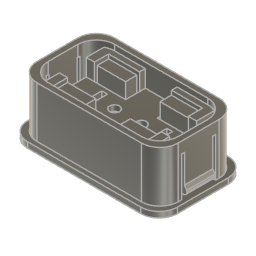
miata-dash-clip (Autodesk Fusion 360 design; units mm, degrees)
Autodesk Fusion 360 part; units mm, degrees
other "Grundnetzelement1"
sketch "Skizze1" plane through (0, 0, 0) normal (0, 0, 1) x (1, 0, 0)
  line L0 (0, 0) -> (53, 0)
  line L1 (53, 0) -> (53, 31)
  line L2 (53, 31) -> (0, 31)
  line L3 (0, 31) -> (0, 0)
  line L4 (1.5, 29.2511) -> (51.4995, 29.2511)
  line L5 (51.4995, 29.2511) -> (51.4995, 1.752)
  line L6 (51.4995, 1.752) -> (1.5, 1.752)
  line L7 (1.5, 1.752) -> (1.5, 29.2511)
  line L8 (49.4995, 27.2511) -> (49.4995, 3.752)
  line L9 (49.4995, 3.752) -> (3.5, 3.752)
  line L10 (3.5, 3.752) -> (3.5, 27.2511)
  line L11 (3.5, 27.2511) -> (49.4995, 27.2511)
  dimension "d1" = 2
  constraint horizontal L0
  constraint vertical L1
  constraint horizontal L2
  constraint vertical L3
  constraint coincident L0.start L3.end
  constraint horizontal L4
  constraint vertical L5
  constraint horizontal L6
  constraint vertical L7
extrude "Extrusion1" add sketch "Skizze1" along normal blind 2 contours L0 L1 L2 L3 | L4 L5 L6 L7 makes body 1
extrude "Extrusion2" add sketch "Skizze1" along normal blind 20 contours L4 L5 L6 L7 bodies 1
fillet "Abrundung1" radius 6.5 12 edges at (51.4995, 29.2511, 11) (53, 31, 1) (53, 0, 1) (51.4995, 1.752, 11) (0, 0, 1) (1.5, 1.752, 11) (0, 31, 1) (1.5, 29.2511, 11) (49.4995, 27.2511, 10) (3.5, 27.2511, 10) (3.5, 3.752, 10) (49.4995, 3.752, 10) on bodies 1
sketch "Skizze2" plane through (51.4995, 0, 0) normal (1, 0, 0) x (0, 1, 0)
  line L0 (8.252, 20) -> (8.252, 2)
  line L1 (8.252, 2) -> (22.7511, 2)
  line L2 (22.7511, 2) -> (22.7511, 20)
  line L3 (22.7511, 20) -> (8.252, 20)
  line L4 (10.5, 16) -> (9.5, 16)
  line L5 (9.5, 16) -> (9.5, 2)
  line L6 (10.5, 16) -> (10.5, 3)
  line L7 (10.5, 3) -> (20.5, 3)
  line L8 (20.5, 3) -> (20.5, 16)
  line L9 (20.5, 16) -> (21.5, 16)
  line L10 (21.5, 16) -> (21.5, 2)
  constraint horizontal L4
  constraint coincident L1 L5.end
  constraint perpendicular L1 L5
  constraint perpendicular L4 L6
  constraint perpendicular L6 L7
  constraint perpendicular L7 L8
  constraint perpendicular L8 L9
  constraint coincident L1 L10.end
  constraint perpendicular L1 L10
extrude "Extrusion3" cut sketch "Skizze2" against normal blind 58 contours L1 L4 L5 L6 L7 L8 L9 L10 bodies 1
sketch "Skizze3" plane through (51.4995, 0, 0) normal (1, 0, 0) x (0, 1, 0)
  line L0 (21.5, 16) -> (21.5, 2)
  line L1 (21.5, 2) -> (22.7511, 2)
  line L2 (22.7511, 2) -> (22.7511, 20)
  line L3 (22.7511, 20) -> (8.252, 20)
  line L4 (8.252, 20) -> (8.252, 2)
  line L5 (8.252, 2) -> (9.5, 2)
  line L6 (9.5, 2) -> (9.5, 16)
  line L7 (9.5, 16) -> (10.5, 16)
  line L8 (10.5, 16) -> (10.5, 3)
  line L9 (10.5, 3) -> (20.5, 3)
  line L10 (20.5, 3) -> (20.5, 16)
  line L11 (20.5, 16) -> (21.5, 16)
  line L12 (10.5, 6) -> (20.5, 6)
  constraint coincident L8 L12.start
  constraint coincident L10 L12.end
  constraint perpendicular L10 L12
extrude "Extrusion4" add sketch "Skizze3" along normal blind 0.9 contours L8 L9 L10 L12 bodies 1
sketch "Skizze4" plane through (1.5, 0, 0) normal (-1, 0, 0) x (0, -1, 0)
  line L0 (-21.5, 2) -> (-21.5, 16)
  line L1 (-21.5, 16) -> (-20.5, 16)
  line L2 (-20.5, 16) -> (-20.5, 3)
  line L3 (-20.5, 3) -> (-10.5, 3)
  line L4 (-10.5, 3) -> (-10.5, 16)
  line L5 (-10.5, 16) -> (-9.5, 16)
  line L6 (-9.5, 16) -> (-9.5, 2)
  line L7 (-9.5, 2) -> (-8.252, 2)
  line L8 (-8.252, 2) -> (-8.252, 20)
  line L9 (-8.252, 20) -> (-22.7511, 20)
  line L10 (-22.7511, 20) -> (-22.7511, 2)
  line L11 (-22.7511, 2) -> (-21.5, 2)
  line L12 (-20.5, 6) -> (-10.5, 6)
  constraint coincident L2 L12.start
  constraint coincident L4 L12.end
  constraint perpendicular L4 L12
extrude "Extrusion5" add sketch "Skizze4" along normal blind 0.9 contours L2 L3 L4 L12 bodies 1
chamfer "Fase1" distance 1.5 distance2 0.9 2 edges at (0.6, 15.5, 6) (52.3995, 15.5, 6) measured on face at (0.6, 17.1667, 5) measured on face at (52.3995, 13.8333, 5) on bodies 1
chamfer "Fase2" distance 0.75 distance2 0.9 2 edges at (52.3995, 15.5, 3) (0.6, 15.5, 3) measured on face at (52.3995, 13.8333, 4.0002) measured on face at (0.6, 17.1667, 3.5001) on bodies 1
fillet "Abrundung2" radius 1 4 edges at (52.3995, 15.5, 4.5) (52.3995, 15.5, 3.75) (0.6, 15.5, 4.5) (0.6, 15.5, 3.75) on bodies 1
sketch "Skizze1 (2)" plane through (0, 0, 0) normal (0, 0, -1) x (1, 0, 0) in component "button-holder"
  arc A0 (0, -24.5) -> (6.5, -31) centre (6.5, -24.5) ccw
  line L0 (6.5, -31) -> (46.5, -31)
  arc A1 (46.5, -31) -> (53, -24.5) centre (46.5, -24.5) ccw
  line L1 (53, -24.5) -> (53, -6.5)
  arc A2 (53, -6.5) -> (46.5, 0) centre (46.5, -6.5) ccw
  line L2 (46.5, 0) -> (6.5, 0)
  arc A3 (6.5, 0) -> (0, -6.5) centre (6.5, -6.5) ccw
  line L3 (0, -6.5) -> (0, -24.5)
  line L4 (7, -31) -> (7, 0)
  line L5 (46, -31) -> (46, 0)
  arc A4 (10, -3.752) -> (3.5, -10.252) centre (10, -10.252) ccw
  line L6 (10, -3.752) -> (42.9995, -3.752)
  arc A5 (49.4995, -10.252) -> (42.9995, -3.752) centre (42.9995, -10.252) ccw
  line L7 (49.4995, -10.252) -> (49.4995, -20.7511)
  arc A6 (42.9995, -27.2511) -> (49.4995, -20.7511) centre (42.9995, -20.7511) ccw
  line L8 (42.9995, -27.2511) -> (10, -27.2511)
  arc A7 (3.5, -20.7511) -> (10, -27.2511) centre (10, -20.7511) ccw
  line L9 (3.5, -20.7511) -> (3.5, -10.252)
  dimension "d20" = 7
  dimension "d21" = 7
  constraint coincident L0 L4.start
  constraint coincident L2 L4.end
  constraint perpendicular L2 L4
  constraint coincident L0 L5.start
  constraint coincident L2 L5.end
  constraint perpendicular L2 L5
  measures "d20" distance of L3 L4
  measures "d21" distance of L1 L5
extrude "Extrusion1'" add sketch "Skizze1 (2)" against normal blind 2 from surface at -10 separate body contours L4 L5 A4 L6 A5 A6 L8 A7 makes body 2 in component "button-holder"
sketch "Skizze2 (2)" plane through (0, 0, 10) normal (0, 0, -1) x (1, 0, 0) in component "button-holder"
  arc A0 (42.9995, -27.2511) -> (46, -26.5172) centre (42.9995, -20.7511) ccw
  line L0 (46, -26.5172) -> (46, -4.486)
  arc A1 (46, -4.486) -> (42.9995, -3.752) centre (42.9995, -10.252) ccw
  line L1 (42.9995, -3.752) -> (10, -3.752)
  arc A2 (10, -3.752) -> (7, -4.4857) centre (10, -10.252) ccw
  line L2 (7, -4.4857) -> (7, -26.5174)
  arc A3 (7, -26.5174) -> (10, -27.2511) centre (10, -20.7511) ccw
  line L3 (10, -27.2511) -> (42.9995, -27.2511)
  line L4 (26.4997, -3.752) -> (26.4997, -27.2511) construction
  arc A4 (10, -3.752) -> (3.5, -10.252) centre (10, -10.252) ccw construction
  line L5 (10, -3.752) -> (42.9995, -3.752) construction
  arc A5 (49.4995, -10.252) -> (42.9995, -3.752) centre (42.9995, -10.252) ccw construction
  line L6 (49.4995, -10.252) -> (49.4995, -20.7511) construction
  arc A6 (42.9995, -27.2511) -> (49.4995, -20.7511) centre (42.9995, -20.7511) ccw construction
  line L7 (42.9995, -27.2511) -> (10, -27.2511) construction
  arc A7 (3.5, -20.7511) -> (10, -27.2511) centre (10, -20.7511) ccw construction
  line L8 (3.5, -20.7511) -> (3.5, -10.252) construction
  arc A8 (0, -24.5) -> (6.5, -31) centre (6.5, -24.5) ccw construction
  line L9 (6.5, -31) -> (46.5, -31) construction
  arc A9 (46.5, -31) -> (53, -24.5) centre (46.5, -24.5) ccw construction
  line L10 (53, -24.5) -> (53, -6.5) construction
  arc A10 (53, -6.5) -> (46.5, 0) centre (46.5, -6.5) ccw construction
  line L11 (46.5, 0) -> (6.5, 0) construction
  arc A11 (6.5, 0) -> (0, -6.5) centre (6.5, -6.5) ccw construction
  line L12 (0, -6.5) -> (0, -24.5) construction
  line L13 (3.5, -15.5016) -> (26.4997, -15.5016) construction
  line L14 (26.4997, -15.5016) -> (49.4995, -15.5016) construction
  line L15 (15.9999, -18.7516) -> (13.9999, -18.7516)
  line L16 (13.9999, -18.7516) -> (13.9999, -12.2516)
  line L17 (13.9999, -12.2516) -> (15.9999, -12.2516)
  line L18 (15.9999, -12.2516) -> (15.9999, -18.7516)
  line L19 (15.9999, -18.7516) -> (13.9999, -12.2516) construction
  line L20 (13.9999, -18.7516) -> (15.9999, -12.2516) construction
  line L21 (38.9996, -18.7516) -> (36.9996, -18.7516)
  line L22 (36.9996, -18.7516) -> (36.9996, -12.2516)
  line L23 (36.9996, -12.2516) -> (38.9996, -12.2516)
  line L24 (38.9996, -12.2516) -> (38.9996, -18.7516)
  line L25 (38.9996, -18.7516) -> (36.9996, -12.2516) construction
  line L26 (36.9996, -18.7516) -> (38.9996, -12.2516) construction
  point P0 (14.9999, -15.5016)
  point P1 (37.9996, -15.5016)
  dimension "d25" = 6.5
  dimension "d26" = 2
  dimension "d27" = 6.5
  dimension "d28" = 2
  constraint midpoint L1 L4.start
  constraint midpoint L3 L4.end
  constraint midpoint L8 L13.start
  constraint midpoint L4 L13.end
  constraint midpoint L6 L14.end
  constraint horizontal L15
  constraint perpendicular L15 L16
  constraint parallel L15 L17
  constraint parallel L16 L18
  constraint coincident L19 P0
  constraint coincident L20 P0
  constraint midpoint L13 P0
  constraint horizontal L21
  constraint perpendicular L21 L22
  constraint parallel L21 L23
  constraint parallel L22 L24
  constraint coincident L25 P1
  constraint coincident L26 P1
  constraint midpoint L14 P1
  measures "d25" distance of L15.end L16.end
  measures "d26" distance of L22.end L23.end
  measures "d27" distance of L21.end L22.end
  measures "d28" distance of L16.end L17.end
extrude "Extrusion2'" cut sketch "Skizze2 (2)" against normal blind 3 contours L15 L16 L17 L18 | L21 L22 L23 L24 bodies 2 in component "button-holder"
sketch "Skizze1 (3)" plane through (0, 0, 0) normal (0, 0, -1) x (1, 0, 0) in component "buttons"
  arc A0 (10, -3.752) -> (3.5, -10.252) centre (10, -10.252) ccw
  line L0 (10, -3.752) -> (42.9995, -3.752)
  arc A1 (49.4995, -10.252) -> (42.9995, -3.752) centre (42.9995, -10.252) ccw
  line L1 (49.4995, -10.252) -> (49.4995, -20.7511)
  arc A2 (42.9995, -27.2511) -> (49.4995, -20.7511) centre (42.9995, -20.7511) ccw
  line L2 (42.9995, -27.2511) -> (10, -27.2511)
  arc A3 (3.5, -20.7511) -> (10, -27.2511) centre (10, -20.7511) ccw
  line L3 (3.5, -20.7511) -> (3.5, -10.252)
  arc A4 (0, -24.5) -> (6.5, -31) centre (6.5, -24.5) ccw
  line L4 (6.5, -31) -> (46.5, -31)
  arc A5 (46.5, -31) -> (53, -24.5) centre (46.5, -24.5) ccw
  line L5 (53, -24.5) -> (53, -6.5)
  arc A6 (53, -6.5) -> (46.5, 0) centre (46.5, -6.5) ccw
  line L6 (46.5, 0) -> (6.5, 0)
  arc A7 (6.5, 0) -> (0, -6.5) centre (6.5, -6.5) ccw
  line L7 (0, -6.5) -> (0, -24.5)
  line L8 (26.4997, -3.752) -> (26.4997, -27.2511) construction
  line L9 (3.5, -15.5016) -> (26.4997, -15.5016) construction
  line L10 (26.4997, -15.5016) -> (49.4995, -15.5016) construction
  line L11 (20.7497, -25.7511) -> (10, -25.7511)
  line L12 (5, -20.7511) -> (5, -10.252)
  line L13 (10, -5.252) -> (20.7497, -5.252)
  line L14 (25.7497, -10.252) -> (25.7497, -20.7511)
  line L15 (42.9995, -25.7511) -> (32.2497, -25.7511)
  line L16 (27.2497, -20.7511) -> (27.2497, -10.252)
  line L17 (32.2497, -5.252) -> (42.9995, -5.252)
  line L18 (47.9995, -10.252) -> (47.9995, -20.7511)
  arc A8 (10, -5.252) -> (5, -10.252) centre (10, -10.252) ccw
  arc A9 (25.7497, -10.252) -> (20.7497, -5.252) centre (20.7497, -10.252) ccw
  arc A10 (5, -20.7511) -> (10, -25.7511) centre (10, -20.7511) ccw
  arc A11 (20.7497, -25.7511) -> (25.7497, -20.7511) centre (20.7497, -20.7511) ccw
  arc A12 (27.2497, -20.7511) -> (32.2497, -25.7511) centre (32.2497, -20.7511) ccw
  arc A13 (32.2497, -5.252) -> (27.2497, -10.252) centre (32.2497, -10.252) ccw
  arc A14 (47.9995, -10.252) -> (42.9995, -5.252) centre (42.9995, -10.252) ccw
  arc A15 (42.9995, -25.7511) -> (47.9995, -20.7511) centre (42.9995, -20.7511) ccw
  point P0 (14.9999, -15.5016)
  point P1 (37.9996, -15.5016)
  dimension "d31" = 1.5
  dimension "d32" = 1.5
  dimension "d33" = 0.75
  dimension "d34" = 1.5
  dimension "d35" = 1.5
  dimension "d36" = 1.5
  dimension "d37" = 0.75
  dimension "d38" = 1.5
  dimension "d39" = 5
  constraint midpoint L0 L8.start
  constraint midpoint L2 L8.end
  constraint midpoint L3 L9.start
  constraint midpoint L8 L9.end
  constraint midpoint L1 L10.end
  constraint horizontal L11
  constraint perpendicular L11 L12
  constraint parallel L11 L13
  constraint parallel L12 L14
  constraint midpoint L9 P0
  constraint horizontal L15
  constraint perpendicular L15 L16
  constraint parallel L15 L17
  constraint parallel L16 L18
  constraint midpoint L10 P1
  constraint tangent L12 A8
  constraint tangent L13 A8
  constraint tangent L13 A9
  constraint tangent L14 A9
  constraint equal A8 A9
  constraint tangent L11 A10
  constraint tangent L12 A10
  constraint equal A8 A10
  constraint tangent L11 A11
  constraint tangent L14 A11
  constraint equal A8 A11
  constraint tangent L15 A12
  constraint tangent L16 A12
  constraint equal A8 A12
  constraint tangent L16 A13
  constraint tangent L17 A13
  constraint equal A8 A13
  constraint tangent L17 A14
  constraint tangent L18 A14
  constraint equal A8 A14
  constraint tangent L15 A15
  constraint tangent L18 A15
  constraint equal A8 A15
  measures "d31" distance of L2 L15
  measures "d32" distance of L1 L18
  measures "d33" distance of L8 L16
  measures "d34" distance of L0 L17
  measures "d35" distance of L0 L13
  measures "d36" distance of L3 L12
  measures "d37" distance of L8 L14
  measures "d38" distance of L2 L11
  measures "d39" radius of A8
extrude "Extrusion1''" add sketch "Skizze1 (3)" against normal blind 8 from surface at 3 separate body contours L11 L12 L13 L14 A8 A9 A10 A11 | L15 L16 L17 L18 A12 A13 A14 A15 makes body 3 at (39.4162, 18.9181, -3) makes body 4 at (17.1665, 18.9181, -3) in component "buttons"
fillet "Abrundung1'" radius 1.5 16 edges at (37.6246, 25.7511, -3) (46.535, 24.2867, -3) (47.9995, 15.5016, -3) (46.535, 6.7165, -3) (37.6246, 5.252, -3) (28.7142, 6.7165, -3) (27.2497, 15.5016, -3) (28.7142, 24.2867, -3) (15.3749, 25.7511, -3) (24.2853, 24.2867, -3) (25.7497, 15.5016, -3) (24.2853, 6.7165, -3) (15.3749, 5.252, -3) (6.4645, 6.7165, -3) (5, 15.5016, -3) (6.4645, 24.2867, -3) on bodies 3 4 in component "buttons"
sketch "Skizze2 (3)" plane through (0, 0, 5) normal (0, 0, 1) x (-1, 0, 0) in component "buttons"
  arc A0 (-10, -25.7511) -> (-5, -20.7511) centre (-10, -20.7511) ccw
  line L0 (-5, -20.7511) -> (-5, -10.252)
  arc A1 (-5, -10.252) -> (-10, -5.252) centre (-10, -10.252) ccw
  line L1 (-10, -5.252) -> (-20.7497, -5.252)
  arc A2 (-20.7497, -5.252) -> (-25.7497, -10.252) centre (-20.7497, -10.252) ccw
  line L2 (-25.7497, -10.252) -> (-25.7497, -20.7511)
  arc A3 (-25.7497, -20.7511) -> (-20.7497, -25.7511) centre (-20.7497, -20.7511) ccw
  line L3 (-20.7497, -25.7511) -> (-10, -25.7511)
  arc A4 (-32.2497, -25.7511) -> (-27.2497, -20.7511) centre (-32.2497, -20.7511) ccw
  line L4 (-27.2497, -20.7511) -> (-27.2497, -10.252)
  arc A5 (-27.2497, -10.252) -> (-32.2497, -5.252) centre (-32.2497, -10.252) ccw
  line L5 (-32.2497, -5.252) -> (-42.9995, -5.252)
  arc A6 (-42.9995, -5.252) -> (-47.9995, -10.252) centre (-42.9995, -10.252) ccw
  line L6 (-47.9995, -10.252) -> (-47.9995, -20.7511)
  arc A7 (-47.9995, -20.7511) -> (-42.9995, -25.7511) centre (-42.9995, -20.7511) ccw
  line L7 (-42.9995, -25.7511) -> (-32.2497, -25.7511)
  line L8 (-10, -3.752) -> (-42.9995, -3.752) construction
  line L9 (-42.9995, -27.2511) -> (-10, -27.2511) construction
  line L10 (-15.3749, -5.252) -> (-15.3749, -25.7511) construction
  line L11 (-37.6246, -5.252) -> (-37.6246, -25.7511) construction
  line L12 (-32.6246, -10.252) -> (-42.6246, -10.252)
  line L13 (-42.6246, -10.252) -> (-42.6246, -6.252)
  line L14 (-42.6246, -6.252) -> (-32.6246, -6.252)
  line L15 (-32.6246, -6.252) -> (-32.6246, -10.252)
  line L16 (-32.6246, -10.252) -> (-42.6246, -6.252) construction
  line L17 (-42.6246, -10.252) -> (-32.6246, -6.252) construction
  line L18 (-10.3749, -10.252) -> (-20.3749, -10.252)
  line L19 (-20.3749, -10.252) -> (-20.3749, -6.252)
  line L20 (-20.3749, -6.252) -> (-10.3749, -6.252)
  line L21 (-10.3749, -6.252) -> (-10.3749, -10.252)
  line L22 (-10.3749, -10.252) -> (-20.3749, -6.252) construction
  line L23 (-20.3749, -10.252) -> (-10.3749, -6.252) construction
  line L24 (-10.3749, -24.7511) -> (-20.3749, -24.7511)
  line L25 (-20.3749, -24.7511) -> (-20.3749, -20.7511)
  line L26 (-20.3749, -20.7511) -> (-10.3749, -20.7511)
  line L27 (-10.3749, -20.7511) -> (-10.3749, -24.7511)
  line L28 (-10.3749, -24.7511) -> (-20.3749, -20.7511) construction
  line L29 (-20.3749, -24.7511) -> (-10.3749, -20.7511) construction
  line L30 (-32.6246, -24.7511) -> (-42.6246, -24.7511)
  line L31 (-42.6246, -24.7511) -> (-42.6246, -20.7511)
  line L32 (-42.6246, -20.7511) -> (-32.6246, -20.7511)
  line L33 (-32.6246, -20.7511) -> (-32.6246, -24.7511)
  line L34 (-32.6246, -24.7511) -> (-42.6246, -20.7511) construction
  line L35 (-42.6246, -24.7511) -> (-32.6246, -20.7511) construction
  point P0 (-37.6246, -8.252)
  point P1 (-15.3749, -8.252)
  point P2 (-15.3749, -22.7511)
  point P3 (-37.6246, -22.7511)
  dimension "d45" = 10
  dimension "d46" = 4
  dimension "d47" = 3
  dimension "d48" = 10
  dimension "d49" = 4
  dimension "d50" = 10
  dimension "d51" = 4
  dimension "d52" = 10
  dimension "d53" = 4
  dimension "d54" = 3
  dimension "d55" = 3
  dimension "d56" = 3
  constraint midpoint L1 L10.start
  constraint midpoint L3 L10.end
  constraint midpoint L5 L11.start
  constraint midpoint L7 L11.end
  constraint horizontal L12
  constraint perpendicular L12 L13
  constraint parallel L12 L14
  constraint parallel L13 L15
  constraint coincident L16 P0
  constraint coincident L17 P0
  constraint coincident L11 P0
  constraint horizontal L18
  constraint perpendicular L18 L19
  constraint parallel L18 L20
  constraint parallel L19 L21
  constraint coincident L22 P1
  constraint coincident L23 P1
  constraint coincident L10 P1
  constraint horizontal L24
  constraint perpendicular L24 L25
  constraint parallel L24 L26
  constraint parallel L25 L27
  constraint coincident L28 P2
  constraint coincident L29 P2
  constraint coincident L10 P2
  constraint horizontal L30
  constraint perpendicular L30 L31
  constraint parallel L30 L32
  constraint parallel L31 L33
  constraint coincident L34 P3
  constraint coincident L35 P3
  constraint coincident L11 P3
  measures "d45" distance of L13.end L14.end
  measures "d46" distance of L12.end L13.end
  measures "d47" distance of L5 P0
  measures "d48" distance of L19.end L20.end
  measures "d49" distance of L18.end L19.end
  measures "d50" distance of L25.end L26.end
  measures "d51" distance of L24.end L25.end
  measures "d52" distance of L31.end L32.end
  measures "d53" distance of L30.end L31.end
  measures "d54" distance of L7 P3
  measures "d55" distance of L3 P2
  measures "d56" distance of L1 P1
extrude "Extrusion2''" add sketch "Skizze2 (3)" along normal blind 12 contours L12 L13 L14 L15 | L18 L19 L20 L21 | L24 L25 L26 L27 | L30 L31 L32 L33 bodies 3 4 in component "buttons"
sketch "Skizze3 (2)" plane through (0, 0, 12) normal (0, 0, 1) x (-1, 0, 0) in component "button-holder"
  line L0 (-13.9999, -12.2516) -> (-13.9999, -18.7516)
  line L1 (-13.9999, -18.7516) -> (-15.9999, -18.7516)
  line L2 (-15.9999, -18.7516) -> (-15.9999, -12.2516)
  line L3 (-15.9999, -12.2516) -> (-13.9999, -12.2516)
  line L4 (-36.9996, -12.2516) -> (-36.9996, -18.7516)
  line L5 (-36.9996, -18.7516) -> (-38.9996, -18.7516)
  line L6 (-38.9996, -18.7516) -> (-38.9996, -12.2516)
  line L7 (-38.9996, -12.2516) -> (-36.9996, -12.2516)
  arc A0 (-46, -26.5172) -> (-42.9995, -27.2511) centre (-42.9995, -20.7511) ccw
  line L8 (-42.9995, -27.2511) -> (-10, -27.2511)
  arc A1 (-10, -27.2511) -> (-7, -26.5174) centre (-10, -20.7511) ccw
  line L9 (-7, -26.5174) -> (-7, -4.4857)
  arc A2 (-7, -4.4857) -> (-10, -3.752) centre (-10, -10.252) ccw
  line L10 (-10, -3.752) -> (-42.9995, -3.752)
  arc A3 (-42.9995, -3.752) -> (-46, -4.486) centre (-42.9995, -10.252) ccw
  line L11 (-46, -4.486) -> (-46, -26.5172)
  line L12 (-10.3749, -6.252) -> (-20.3749, -6.252)
  line L13 (-20.3749, -6.252) -> (-20.3749, -10.252)
  line L14 (-20.3749, -10.252) -> (-10.3749, -10.252)
  line L15 (-10.3749, -10.252) -> (-10.3749, -6.252)
  line L16 (-32.6246, -6.252) -> (-42.6246, -6.252)
  line L17 (-42.6246, -6.252) -> (-42.6246, -10.252)
  line L18 (-42.6246, -10.252) -> (-32.6246, -10.252)
  line L19 (-32.6246, -10.252) -> (-32.6246, -6.252)
  line L20 (-32.6246, -20.7511) -> (-42.6246, -20.7511)
  line L21 (-42.6246, -20.7511) -> (-42.6246, -24.7511)
  line L22 (-42.6246, -24.7511) -> (-32.6246, -24.7511)
  line L23 (-32.6246, -24.7511) -> (-32.6246, -20.7511)
  line L24 (-10.3749, -20.7511) -> (-20.3749, -20.7511)
  line L25 (-20.3749, -20.7511) -> (-20.3749, -24.7511)
  line L26 (-20.3749, -24.7511) -> (-10.3749, -24.7511)
  line L27 (-10.3749, -24.7511) -> (-10.3749, -20.7511)
  line L28 (-32.1246, -5.752) -> (-43.1246, -5.752)
  line L29 (-43.1246, -5.752) -> (-43.1246, -10.752)
  line L30 (-43.1246, -10.752) -> (-32.1246, -10.752)
  line L31 (-32.1246, -10.752) -> (-32.1246, -5.752)
  line L32 (-9.8749, -5.752) -> (-20.8749, -5.752)
  line L33 (-20.8749, -5.752) -> (-20.8749, -10.752)
  line L34 (-20.8749, -10.752) -> (-9.8749, -10.752)
  line L35 (-9.8749, -10.752) -> (-9.8749, -5.752)
  line L36 (-9.8749, -20.2511) -> (-20.8749, -20.2511)
  line L37 (-20.8749, -20.2511) -> (-20.8749, -25.2511)
  line L38 (-20.8749, -25.2511) -> (-9.8749, -25.2511)
  line L39 (-9.8749, -25.2511) -> (-9.8749, -20.2511)
  line L40 (-32.1246, -20.2511) -> (-43.1246, -20.2511)
  line L41 (-43.1246, -20.2511) -> (-43.1246, -25.2511)
  line L42 (-43.1246, -25.2511) -> (-32.1246, -25.2511)
  line L43 (-32.1246, -25.2511) -> (-32.1246, -20.2511)
  line L44 (-20.8749, -5.752) -> (-20.8749, -3.752)
  line L45 (-9.8749, -10.752) -> (-7, -10.752)
  line L46 (-9.8749, -20.2511) -> (-7, -20.2511)
  line L47 (-20.8749, -25.2511) -> (-20.8749, -27.2511)
  line L48 (-32.1246, -25.2511) -> (-32.1246, -27.2511)
  line L49 (-43.1246, -20.2511) -> (-46, -20.2511)
  line L50 (-43.1246, -10.752) -> (-46, -10.752)
  line L51 (-32.1246, -5.752) -> (-32.1246, -3.752)
  dimension "d59" = 0.5
  dimension "d60" = 0.5
  dimension "d61" = 0.5
  dimension "d62" = 0.5
  constraint coincident L10 L44.end
  constraint perpendicular L10 L44
  constraint coincident L9 L45.end
  constraint perpendicular L9 L45
  constraint coincident L9 L46.end
  constraint perpendicular L9 L46
  constraint coincident L8 L47.end
  constraint perpendicular L8 L47
  constraint coincident L8 L48.end
  constraint perpendicular L8 L48
  constraint perpendicular L11 L49
  constraint perpendicular L11 L50
  constraint coincident L10 L51.end
  constraint perpendicular L10 L51
extrude "Extrusion3'" cut sketch "Skizze3 (2)" against normal blind 4 contours L40 L41 L42 L43 | L28 L29 L30 L31 | L36 L37 L38 L39 | L32 L33 L34 L35 | L12 L13 L14 L15 | L16 L17 L18 L19 | L20 L21 L22 L23 | L24 L25 L26 L27 bodies 2 in component "button-holder"
sketch "Skizze5" plane through (0, 0, 0) normal (0, 0, -1) x (1, 0, 0)
  arc A0 (10, -3.752) -> (3.5, -10.252) centre (10, -10.252) ccw
  line L0 (10, -3.752) -> (42.9995, -3.752)
  arc A1 (49.4995, -10.252) -> (42.9995, -3.752) centre (42.9995, -10.252) ccw
  line L1 (49.4995, -10.252) -> (49.4995, -20.7511)
  arc A2 (42.9995, -27.2511) -> (49.4995, -20.7511) centre (42.9995, -20.7511) ccw
  line L2 (42.9995, -27.2511) -> (10, -27.2511)
  arc A3 (3.5, -20.7511) -> (10, -27.2511) centre (10, -20.7511) ccw
  line L3 (3.5, -20.7511) -> (3.5, -10.252)
  arc A4 (0, -24.5) -> (6.5, -31) centre (6.5, -24.5) ccw
  line L4 (6.5, -31) -> (46.5, -31)
  arc A5 (46.5, -31) -> (53, -24.5) centre (46.5, -24.5) ccw
  line L5 (53, -24.5) -> (53, -6.5)
  arc A6 (53, -6.5) -> (46.5, 0) centre (46.5, -6.5) ccw
  line L6 (46.5, 0) -> (6.5, 0)
  arc A7 (6.5, 0) -> (0, -6.5) centre (6.5, -6.5) ccw
  line L7 (0, -6.5) -> (0, -24.5)
  arc A8 (25.7497, -10.252) -> (20.7497, -5.252) centre (20.7497, -10.252) ccw
  line L8 (25.7497, -10.252) -> (25.7497, -20.7511)
  arc A9 (20.7497, -25.7511) -> (25.7497, -20.7511) centre (20.7497, -20.7511) ccw
  line L9 (20.7497, -25.7511) -> (10, -25.7511)
  line L10 (10, -5.252) -> (20.7497, -5.252)
  arc A10 (10, -5.252) -> (5, -10.252) centre (10, -10.252) ccw
  line L11 (5, -20.7511) -> (5, -10.252)
  arc A11 (5, -20.7511) -> (10, -25.7511) centre (10, -20.7511) ccw
  arc A12 (47.9995, -10.252) -> (42.9995, -5.252) centre (42.9995, -10.252) ccw
  line L12 (47.9995, -10.252) -> (47.9995, -20.7511)
  arc A13 (42.9995, -25.7511) -> (47.9995, -20.7511) centre (42.9995, -20.7511) ccw
  line L13 (42.9995, -25.7511) -> (32.2497, -25.7511)
  line L14 (32.2497, -5.252) -> (42.9995, -5.252)
  arc A14 (32.2497, -5.252) -> (27.2497, -10.252) centre (32.2497, -10.252) ccw
  line L15 (27.2497, -20.7511) -> (27.2497, -10.252)
  arc A15 (27.2497, -20.7511) -> (32.2497, -25.7511) centre (32.2497, -20.7511) ccw
  line L16 (42.9995, -26.5511) -> (32.2497, -26.5511)
  arc A16 (26.4497, -20.7511) -> (32.2497, -26.5511) centre (32.2497, -20.7511) ccw
  line L17 (26.4497, -20.7511) -> (26.4497, -10.252)
  arc A17 (32.2497, -4.452) -> (26.4497, -10.252) centre (32.2497, -10.252) ccw
  line L18 (32.2497, -4.452) -> (42.9995, -4.452)
  arc A18 (48.7995, -10.252) -> (42.9995, -4.452) centre (42.9995, -10.252) ccw
  line L19 (48.7995, -10.252) -> (48.7995, -20.7511)
  arc A19 (42.9995, -26.5511) -> (48.7995, -20.7511) centre (42.9995, -20.7511) ccw
  arc A20 (4.2, -20.7511) -> (10, -26.5511) centre (10, -20.7511) ccw
  line L20 (20.7497, -26.5511) -> (10, -26.5511)
  arc A21 (20.7497, -26.5511) -> (26.5497, -20.7511) centre (20.7497, -20.7511) ccw
  line L21 (26.5497, -10.252) -> (26.5497, -20.7511)
  arc A22 (26.5497, -10.252) -> (20.7497, -4.452) centre (20.7497, -10.252) ccw
  line L22 (10, -4.452) -> (20.7497, -4.452)
  arc A23 (10, -4.452) -> (4.2, -10.252) centre (10, -10.252) ccw
  line L23 (4.2, -20.7511) -> (4.2, -10.252)
  dimension "d65" = 0.8
  dimension "d66" = -0.8
extrude "Extrusion6" add sketch "Skizze5" against normal blind 2 contours A0 L0 A1 L1 A2 L2 A3 L3 bodies 1
fillet "Abrundung3" radius 1 2 edges at (26.4997, 9.4921, 1) (26.4997, 21.5111, 1) on bodies 1
sketch "Skizze4 (2)" plane through (0, 0, 12) normal (0, 0, 1) x (-1, 0, 0) in component "buttons"
  line L0 (-20.8749, -20.2511) -> (-9.8749, -20.2511)
  line L1 (-9.8749, -20.2511) -> (-9.8749, -25.2511)
  line L2 (-9.8749, -25.2511) -> (-20.8749, -25.2511)
  line L3 (-20.8749, -25.2511) -> (-20.8749, -20.2511)
  line L4 (-43.1246, -20.2511) -> (-32.1246, -20.2511)
  line L5 (-32.1246, -20.2511) -> (-32.1246, -25.2511)
  line L6 (-32.1246, -25.2511) -> (-43.1246, -25.2511)
  line L7 (-43.1246, -25.2511) -> (-43.1246, -20.2511)
  line L8 (-20.8749, -5.752) -> (-9.8749, -5.752)
  line L9 (-9.8749, -5.752) -> (-9.8749, -10.752)
  line L10 (-9.8749, -10.752) -> (-20.8749, -10.752)
  line L11 (-20.8749, -10.752) -> (-20.8749, -5.752)
  line L12 (-43.1246, -5.752) -> (-32.1246, -5.752)
  line L13 (-32.1246, -5.752) -> (-32.1246, -10.752)
  line L14 (-32.1246, -10.752) -> (-43.1246, -10.752)
  line L15 (-43.1246, -10.752) -> (-43.1246, -5.752)
  line L16 (-13.9999, -12.2516) -> (-13.9999, -18.7516)
  line L17 (-13.9999, -18.7516) -> (-15.9999, -18.7516)
  line L18 (-15.9999, -18.7516) -> (-15.9999, -12.2516)
  line L19 (-15.9999, -12.2516) -> (-13.9999, -12.2516)
  line L20 (-36.9996, -12.2516) -> (-36.9996, -18.7516)
  line L21 (-36.9996, -18.7516) -> (-38.9996, -18.7516)
  line L22 (-38.9996, -18.7516) -> (-38.9996, -12.2516)
  line L23 (-38.9996, -12.2516) -> (-36.9996, -12.2516)
  arc A0 (-46, -26.5172) -> (-42.9995, -27.2511) centre (-42.9995, -20.7511) ccw
  line L24 (-42.9995, -27.2511) -> (-10, -27.2511)
  arc A1 (-10, -27.2511) -> (-7, -26.5174) centre (-10, -20.7511) ccw
  line L25 (-7, -26.5174) -> (-7, -4.4857)
  arc A2 (-7, -4.4857) -> (-10, -3.752) centre (-10, -10.252) ccw
  line L26 (-10, -3.752) -> (-42.9995, -3.752)
  arc A3 (-42.9995, -3.752) -> (-46, -4.486) centre (-42.9995, -10.252) ccw
  line L27 (-46, -4.486) -> (-46, -26.5172)
  line L28 (-32.6246, -6.252) -> (-32.6246, -10.252)
  line L29 (-32.6246, -10.252) -> (-42.6246, -10.252)
  line L30 (-42.6246, -10.252) -> (-42.6246, -6.252)
  line L31 (-42.6246, -6.252) -> (-32.6246, -6.252)
  line L32 (-32.6246, -20.7511) -> (-32.6246, -24.7511)
  line L33 (-32.6246, -24.7511) -> (-42.6246, -24.7511)
  line L34 (-42.6246, -24.7511) -> (-42.6246, -20.7511)
  line L35 (-42.6246, -20.7511) -> (-32.6246, -20.7511)
  arc A4 (-32.2497, -25.7511) -> (-27.2497, -20.7511) centre (-32.2497, -20.7511) ccw
  line L36 (-27.2497, -20.7511) -> (-27.2497, -10.252)
  arc A5 (-27.2497, -10.252) -> (-32.2497, -5.252) centre (-32.2497, -10.252) ccw
  line L37 (-32.2497, -5.252) -> (-42.9995, -5.252)
  arc A6 (-42.9995, -5.252) -> (-47.9995, -10.252) centre (-42.9995, -10.252) ccw
  line L38 (-47.9995, -10.252) -> (-47.9995, -20.7511)
  arc A7 (-47.9995, -20.7511) -> (-42.9995, -25.7511) centre (-42.9995, -20.7511) ccw
  line L39 (-42.9995, -25.7511) -> (-32.2497, -25.7511)
  line L40 (-10.3749, -20.7511) -> (-10.3749, -24.7511)
  line L41 (-10.3749, -24.7511) -> (-20.3749, -24.7511)
  line L42 (-20.3749, -24.7511) -> (-20.3749, -20.7511)
  line L43 (-20.3749, -20.7511) -> (-10.3749, -20.7511)
  line L44 (-10.3749, -6.252) -> (-10.3749, -10.252)
  line L45 (-10.3749, -10.252) -> (-20.3749, -10.252)
  line L46 (-20.3749, -10.252) -> (-20.3749, -6.252)
  line L47 (-20.3749, -6.252) -> (-10.3749, -6.252)
  arc A8 (-10, -25.7511) -> (-5, -20.7511) centre (-10, -20.7511) ccw
  line L48 (-5, -20.7511) -> (-5, -10.252)
  arc A9 (-5, -10.252) -> (-10, -5.252) centre (-10, -10.252) ccw
  line L49 (-10, -5.252) -> (-20.7497, -5.252)
  arc A10 (-20.7497, -5.252) -> (-25.7497, -10.252) centre (-20.7497, -10.252) ccw
  line L50 (-25.7497, -10.252) -> (-25.7497, -20.7511)
  arc A11 (-25.7497, -20.7511) -> (-20.7497, -25.7511) centre (-20.7497, -20.7511) ccw
  line L51 (-20.7497, -25.7511) -> (-10, -25.7511)
  line L52 (-27.2497, -15.5016) -> (-31.2497, -15.5016) construction
  line L53 (-25.7497, -15.5016) -> (-21.7497, -15.5016) construction
  circle A12 centre (-31.2497, -15.5016) radius 1
  circle A13 centre (-21.7497, -15.5016) radius 1
  circle A14 centre (-21.7497, -15.5016) radius 1.75
  circle A15 centre (-31.2497, -15.5016) radius 1.75
  dimension "d73" = 4
  dimension "d74" = 4
  dimension "d75" = 2
  dimension "d76" = 2
  dimension "d77" = 3.5
  dimension "d78" = 3.5
  constraint midpoint L36 L52.start
  constraint perpendicular L36 L52
  constraint midpoint L50 L53.start
  constraint perpendicular L50 L53
  constraint coincident L52.end A12.centre
  constraint coincident L53.end A13.centre
  constraint concentric A13 A14
  constraint concentric A12 A15
  measures "d73" distance of L52.start L52.end
  measures "d74" distance of L53.start L53.end
  measures "d75" diameter of A12
  measures "d76" diameter of A13
  measures "d77" diameter of A14
  measures "d78" diameter of A15
extrude "Extrusion6'" add sketch "Skizze3 (2)" along normal blind 6 contours A0 L8 L11 L41 L42 L48 L49 | L10 A3 L11 L28 L29 L50 L51 | L8 A1 L9 L38 L39 L46 L47 | L9 A2 L10 L32 L35 L44 L45 bodies 2 in component "button-holder"
extrude "Extrusion4'" cut sketch "Skizze4 (2)" against normal blind 12 contours A12 | A13 bodies 2 in component "button-holder"
extrude "Extrusion3''" cut sketch "Skizze4 (2)" against normal blind 12 contours A12 | A13 bodies 3 4 in component "buttons"
extrude "Extrusion5'" cut sketch "Skizze4 (2)" against normal blind 3 contours A14 | A15 bodies 2 in component "button-holder"
combine "Kombinieren1" operation add target body 2 tool bodies 1 in component "button-holder"
component "button-holder" placed x (1, 0, 0) y (0, 1, 0) z (0, 0, 1) at (0, 0, 0)
component "buttons" placed x (1, 0, 0) y (0, 1, 0) z (0, 0, 1) at (0, 0, 0)
equation "d33 = 1.50 mm / 2"
equation "d37 = ( 1.5 / 2 ) * 1 mm"
equation "d40 = -13.00 mm + 5 mm"
